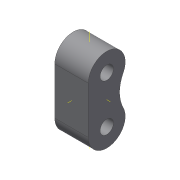
# Autodesk Inventor part: empty
Saved by Autodesk Inventor 2014 (Build 180170000, 170)
## iProperties
Created: 2015-04-13
Part Number: empty
Material: Generic
Document SubType Name: Modeling
Designer: Martin
Density: 1 g/cm^3
Appearance: Default
Author: Martin
Autodesk Inventor part; units mm, degrees
ref_plane "YZ Plane" through (0, 0, 0) normal (1, 0, 0) x (0, 1, 0)
ref_plane "XZ Plane" through (0, 0, 0) normal (0, 1, 0) x (-1, 0, 0)
ref_plane "XY Plane" through (0, 0, 0) normal (0, 0, 1) x (1, 0, 0)
sketch "Sketch1" plane through (0, 0, 0) normal (1, 0, 0) x (0, 1, 0)
  line L0 (0, -8.75) -> (0, 8.75) projected
  line L1 (-3.85, 0) -> (3.85, 0) projected
  circle A0 centre (0, 3.25) radius 1
  circle A1 centre (0, -3.25) radius 1
  circle A2 centre (0, 3.25) radius 2.75 construction
  circle A3 centre (0, -3.25) radius 2.75 construction
  line L2 (-2.75, 3.25) -> (-2.75, -3.25)
  line L3 (2.75, 3.25) -> (2.75, -3.25)
  arc A4 (2.75, 3.25) -> (-2.75, 3.25) centre (0, 3.25) ccw
  arc A5 (-2.75, -3.25) -> (2.75, -3.25) centre (0, -3.25) ccw
  point P0 (0, 0)
  dimension "d0" = 2
  dimension "d1" = 5.5
  dimension "d2" = 6.5
  constraints: 8 point on circle, 6 centre point, 6 tangent, 4 end point, 2 coincident, 2 equal radius, 2 point on line, 1 parallel, 1 perpendicular, 1 symmetric about line
  measures "d0" diameter of A1
  measures "d1" diameter of A3
  measures "d2" distance of A0.centre A1.centre
extrude "ext_main" add sketch "Sketch1" along normal mid plane 5 contours A5 L2 L1 L0 A1 | L0 A1 L1 L3 A5 | L2 A4 L0 A0 L1 | L1 L0 A0 A4 L3
sketch "Sketch2" plane through (-2.5, 0, 0) normal (-1, 0, 0) x (0, 0, 1)
  arc A0 (3.25, -2.75) -> (3.25, 2.75) centre (3.25, 0) ccw projected
  line L0 (3.25, 2.75) -> (-3.25, 2.75) projected
  arc A1 (-3.25, 2.75) -> (-3.25, -2.75) centre (-3.25, 0) ccw projected
  circle A2 centre (-3.25, 0) radius 2.75
  circle A3 centre (3.25, 0) radius 2.75
  arc A4 (-2.0968, 2.4965) -> (2.0968, 2.4965) centre (0, 7.0356) ccw
  line L1 (-3.25, 2.75) -> (3.25, 2.75)
  point P0 (0, 0)
  dimension "d5" = 5
  constraints: 6 point on circle, 3 centre point, 2 coincident, 2 concentric, 2 end point, 2 point on line, 2 tangent
  measures "d5" radius of A4
extrude "ext_cutaway" cut sketch "Sketch2" against normal through all contours A4 A2 L0 A3
equation "\"d0\" = screw_m2_bore_selfthreading"
equation "\"d1\" = general_bore_smallersupport_diameter"
equation "\"d2\" = clevislink_effective_length"
equation "\"d3\" = clevislink_thickness"
equation "\"screw_m2_bore_selfthreading\" = 2"
equation "\"general_bore_smallersupport_diameter\" = 5.5"
equation "\"clevislink_effective_length\" = 6.5"
equation "\"clevislink_thickness\" = 5"
body "Solid1"
